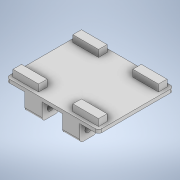
# Autodesk Inventor part: нижняя защелка пушки
Saved by Autodesk Inventor 2020.1 (Build 241239000, 239)
## iProperties
Created: 2022-04-03
Part Number: нижняя защелка пушки
Material: Типовые
Document SubType Name: Modeling
Designer: User
Density: 1 g/cm^3
Appearance: По умолчанию
Author: User
Autodesk Inventor part; units mm, degrees
ref_plane "YZ Plane" through (0, 0, 0) normal (1, 0, 0) x (0, 1, 0)
ref_plane "XZ Plane" through (0, 0, 0) normal (0, 1, 0) x (-1, 0, 0)
ref_plane "XY Plane" through (0, 0, 0) normal (0, 0, 1) x (1, 0, 0)
sketch "Эскиз1" plane through (0, 0, 0) normal (0, 1, 0) x (-1, 0, 0)
  line L0 (0, 0) -> (-25, 0)
  line L1 (-25, 0) -> (-25, 20)
  line L2 (-25, 20) -> (0, 20)
  line L3 (0, 20) -> (0, 0)
  dimension "d0" = 25
  dimension "d1" = 20
  constraints: 8 end point, 2 parallel, 1 horizontal, 1 perpendicular
  measures "d0" distance of L0.start L0.end
  measures "d1" distance of L2.end L0.start
extrude "Выдавливание1" add sketch "Эскиз1" along normal blind 2
sketch "Эскиз2" plane through (0, 2, 0) normal (0, 1, 0) x (1, 0, 0)
  line L0 (25, -20) -> (25, 0) projected
  line L1 (25, 0) -> (10, 0)
  line L2 (10, 0) -> (10, -5)
  line L3 (10, -5) -> (25, -5)
  line L4 (25, -5) -> (25, 0)
  point P0 (0, 0)
  dimension "d4" = 15
  dimension "d5" = 5
  constraints: 8 end point, 2 parallel, 1 horizontal, 1 perpendicular
  measures "d4" distance of L2.end L3.end
  measures "d5" distance of L1.end L2.end
extrude "Выдавливание2" add sketch "Эскиз2" along normal blind 4
mirror "Зеркальное отражение1" about plane through (0, 0, 20) normal (0, 0, 1)
mirror "Зеркальное отражение2" about plane through (0, 0, 0) normal (-1, 0, 0)
sketch "Эскиз3" plane through (0, 2, 0) normal (0, 1, 0) x (1, 0, 0)
  line L0 (-27, 2) -> (27, 2)
  line L1 (27, 2) -> (27, -42)
  line L2 (27, -42) -> (-27, -42)
  line L3 (-27, -42) -> (-27, 2)
  line L4 (25, -5) -> (25, -35) projected
  line L5 (25, 0) -> (10, 0) projected
  line L6 (-25, -5) -> (-25, -35) projected
  line L7 (-10, -40) -> (10, -40) projected
  point P0 (0, 0)
  dimension "d8" = 2
  dimension "d9" = 2
  dimension "d10" = 2
  dimension "d11" = 2
  constraints: 8 end point, 2 parallel, 1 horizontal, 1 perpendicular
  measures "d8" distance between parallel lines of L1 L4
  measures "d9" distance between parallel lines of L0 L5
  measures "d10" distance between parallel lines of L3 L6
  measures "d11" distance between parallel lines of L7 L2
extrude "Выдавливание3" add sketch "Эскиз3" against normal blind 2
sketch "Эскиз4" plane through (0, 0, 0) normal (0, -1, 0) x (1, 0, 0)
  line L0 (27, 42) -> (-27, 42) projected
  line L1 (-27, 42) -> (27, 42)
  line L2 (27, 42) -> (27, 32)
  line L3 (27, 32) -> (-27, 32)
  line L4 (-27, 32) -> (-27, 42)
  line L5 (-27, -2) -> (27, -2) projected
  line L6 (-27, -2) -> (-27, 42) projected
  line L7 (27, -2) -> (-27, -2)
  line L8 (-27, -2) -> (-27, 8)
  line L9 (-27, 8) -> (27, 8)
  line L10 (27, 8) -> (27, -2)
  point P0 (0, 0)
  dimension "d14" = 10
  dimension "d31" = 10
  constraints: 16 end point, 4 parallel, 2 horizontal, 2 perpendicular, 1 point on line
  measures "d14" distance between parallel lines of L0 L3
  measures "d31" distance of L5.end L9.end
extrude "Выдавливание4" add sketch "Эскиз4" along normal blind 10
sketch "Эскиз5" plane through (27, 2, 42) normal (1, 0, 0) x (0, 0, -1)
  line L0 (10, -2) -> (10, -12) projected
  line L1 (0, -12) -> (10, -12) projected
  circle A0 centre (5, -7) radius 2
  line L2 (34, -12) -> (44, -12) projected
  circle A1 centre (39, -7) radius 2
  point P0 (42, -2)
  point P1 (10, -7)
  point P2 (5, -12)
  point P3 (39, -12)
  dimension "d17" = 4
  constraints: 3 midpoint, 2 centre point, 1 equal radius
  measures "d17" diameter of A0
extrude "Выдавливание5" cut sketch "Эскиз5" against normal blind 100
fillet "Сопряжение1" radius 2 4 edges at (0, -10, 42) (0, -10, 32) (0, -10, -2) (0, -10, 8)
sketch "Эскиз6" plane through (0, -10, 0) normal (0, -1, 0) x (1, 0, 0)
  line L0 (27, 32) -> (-27, 32) projected
  line L1 (-27, 42) -> (27, 42) projected
  line L2 (-6, 32) -> (6, 32)
  line L3 (6, 32) -> (6, 42)
  line L4 (6, 42) -> (-6, 42)
  line L5 (-6, 42) -> (-6, 32)
  line L6 (16, 32) -> (31, 32)
  line L7 (31, 32) -> (31, 42)
  line L8 (31, 42) -> (16, 42)
  line L9 (16, 42) -> (16, 32)
  line L10 (-16, 32) -> (-31, 32)
  line L11 (-31, 32) -> (-31, 42)
  line L12 (-31, 42) -> (-16, 42)
  line L13 (-16, 42) -> (-16, 32)
  line L14 (-27, 40) -> (27, 40) projected
  line L15 (0, 40) -> (0, 34)
  line L16 (27, 34) -> (-27, 34) projected
  line L17 (-27, 8) -> (27, 8) projected
  line L18 (16, 8) -> (31, 8)
  line L19 (31, 8) -> (31, -2)
  line L20 (31, -2) -> (16, -2)
  line L21 (16, -2) -> (16, 8)
  line L22 (27, -2) -> (-27, -2) projected
  line L23 (6, 8) -> (-6, 8)
  line L24 (-6, 8) -> (-6, -2)
  line L25 (-6, -2) -> (6, -2)
  line L26 (6, -2) -> (6, 8)
  line L27 (-16, -2) -> (-31, -2)
  line L28 (-31, -2) -> (-31, 8)
  line L29 (-31, 8) -> (-16, 8)
  line L30 (-16, 8) -> (-16, -2)
  point P0 (0, 0)
  dimension "d21" = 15
  dimension "d22" = 15
  dimension "d23" = 12
  dimension "d24" = 10
  dimension "d26" = 10
  constraints: 50 end point, 12 parallel, 11 point on line, 6 horizontal, 6 perpendicular, 2 midpoint, 1 other
  measures "d21" distance of L6.end L6.start
  measures "d22" distance of L10.end L10.start
  measures "d23" distance of L2.end L2.start
  measures "d24" distance of L2.start L10.start
  measures "d26" distance of L6.start L2.end
extrude "Выдавливание6" cut sketch "Эскиз6" against normal blind 10 contours L0 L9 L1 L8 L7 L6 | L0 L5 L16 L3 | L16 L15 L14 L3 | L0 L10 L11 L12 L1 L13 | L5 L14 L15 L16 | L14 L5 L1 L3 | L17 L30 L22 L27 L28 L29 | L17 L26 L22 L24 | L17 L18 L19 L20 L21
fillet "Сопряжение2" radius 2 4 edges at (-27, 1, 42) (27, 1, 42) (-27, 1, -2) (27, 1, -2)
